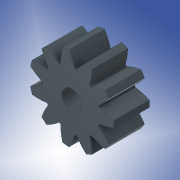
# Autodesk Inventor part: Motor Gear
Saved by Autodesk Inventor 2017 (Build 210142000, 142)
## iProperties
Created: 2017-07-05
Part Number: Motor Gear
Material: ABS Plastic
Document SubType Name: Modeling
Designer: zallen
Density: 1.06 g/cm^3
Appearance: CR Dark Blue
Author: zallen
Autodesk Inventor part; units mm, degrees
ref_plane "YZ Plane" through (0, 0, 0) normal (1, 0, 0) x (0, 1, 0)
ref_plane "XZ Plane" through (0, 0, 0) normal (0, 1, 0) x (-1, 0, 0)
ref_plane "XY Plane" through (0, 0, 0) normal (0, 0, 1) x (1, 0, 0)
sketch "Sketch1" plane through (0, 0, 0) normal (0, 0, 1) x (1, 0, 0)
  circle A0 centre (0, 0) radius 8
  line L0 (0, 0) -> (16, 0) construction
  arc A1 (11.746, 0.9) -> (7.746, 2) centre (5.8068, -12.8741) ccw
  arc A2 (7.746, -2) -> (11.746, -0.9) centre (5.8068, 12.8741) ccw
  arc A3 (7.746, -2) -> (7.746, 2) centre (0, 0) ccw
  arc A4 (11.746, -0.9) -> (11.746, 0.9) centre (-8.2338, 0) ccw
  arc A5 (9.3948, 7.1075) -> (5.435, 5.8703) centre (11.8453, -7.691) ccw
  arc A6 (10.3679, 5.5932) -> (9.3948, 7.1075) centre (-6.9267, -4.4515) ccw
  arc A7 (7.5976, 2.5053) -> (10.3679, 5.5932) centre (-2.0753, 13.9698) ccw
  arc A8 (7.5976, 2.5053) -> (5.435, 5.8703) centre (0, 0) ccw
  arc A9 (4.0608, 11.0584) -> (1.3985, 7.8768) centre (14.123, -0.066) ccw
  arc A10 (5.6981, 10.3106) -> (4.0608, 11.0584) centre (-3.4204, -7.4897) ccw
  arc A11 (5.0371, 6.2151) -> (5.6981, 10.3106) centre (-9.2985, 10.6302) ccw
  arc A12 (5.0371, 6.2151) -> (1.3985, 7.8768) centre (0, 0) ccw
  arc A13 (-2.5625, 11.4983) -> (-3.082, 7.3825) centre (11.9167, 7.5799) ccw
  arc A14 (-0.7808, 11.7545) -> (-2.5625, 11.4983) centre (1.1718, -8.15) ccw
  arc A15 (0.8773, 7.9518) -> (-0.7808, 11.7545) centre (-13.5695, 3.9155) ccw
  arc A16 (0.8773, 7.9518) -> (-3.082, 7.3825) centre (0, 0) ccw
  arc A17 (-8.3721, 8.2876) -> (-6.584, 4.5443) centre (5.927, 12.8193) ccw
  arc A18 (-7.0118, 9.4664) -> (-8.3721, 8.2876) centre (5.392, -6.2227) ccw
  arc A19 (-3.561, 7.1637) -> (-7.0118, 9.4664) centre (-13.5323, -4.0423) ccw
  arc A20 (-3.561, 7.1637) -> (-6.584, 4.5443) centre (0, 0) ccw
  arc A21 (-11.5237, 2.4457) -> (-7.9957, 0.2633) centre (-1.9446, 13.9886) ccw
  arc A22 (-11.0166, 4.1728) -> (-11.5237, 2.4457) centre (7.9002, -2.3197) ccw
  arc A23 (-6.8687, 4.1013) -> (-11.0166, 4.1728) centre (-9.1987, -10.7167) ccw
  arc A24 (-6.8687, 4.1013) -> (-7.9957, 0.2633) centre (0, 0) ccw
  arc A25 (-11.0166, -4.1728) -> (-6.8687, -4.1013) centre (-9.1987, 10.7167) ccw
  arc A26 (-11.5237, -2.4457) -> (-11.0166, -4.1728) centre (7.9002, 2.3197) ccw
  arc A27 (-7.9957, -0.2633) -> (-11.5237, -2.4457) centre (-1.9446, -13.9886) ccw
  arc A28 (-7.9957, -0.2633) -> (-6.8687, -4.1013) centre (0, 0) ccw
  arc A29 (-7.0118, -9.4664) -> (-3.561, -7.1637) centre (-13.5323, 4.0423) ccw
  arc A30 (-8.3721, -8.2876) -> (-7.0118, -9.4664) centre (5.392, 6.2227) ccw
  arc A31 (-6.584, -4.5443) -> (-8.3721, -8.2876) centre (5.927, -12.8193) ccw
  arc A32 (-6.584, -4.5443) -> (-3.561, -7.1637) centre (0, 0) ccw
  arc A33 (-0.7808, -11.7545) -> (0.8773, -7.9518) centre (-13.5695, -3.9155) ccw
  arc A34 (-2.5625, -11.4983) -> (-0.7808, -11.7545) centre (1.1718, 8.15) ccw
  arc A35 (-3.082, -7.3825) -> (-2.5625, -11.4983) centre (11.9167, -7.5799) ccw
  arc A36 (-3.082, -7.3825) -> (0.8773, -7.9518) centre (0, 0) ccw
  arc A37 (5.6981, -10.3106) -> (5.0371, -6.2151) centre (-9.2985, -10.6302) ccw
  arc A38 (4.0608, -11.0584) -> (5.6981, -10.3106) centre (-3.4204, 7.4897) ccw
  arc A39 (1.3985, -7.8768) -> (4.0608, -11.0584) centre (14.123, 0.066) ccw
  arc A40 (1.3985, -7.8768) -> (5.0371, -6.2151) centre (0, 0) ccw
  arc A41 (10.3679, -5.5932) -> (7.5976, -2.5053) centre (-2.0753, -13.9698) ccw
  arc A42 (9.3948, -7.1075) -> (10.3679, -5.5932) centre (-6.9267, 4.4515) ccw
  arc A43 (5.435, -5.8703) -> (9.3948, -7.1075) centre (11.8453, 7.691) ccw
  arc A44 (5.435, -5.8703) -> (7.5976, -2.5053) centre (0, 0) ccw
  point P0 (11.7662, 0)
  point P1 (9.8984, 6.3613)
  point P2 (4.8879, 10.7029)
  point P3 (-1.6745, 11.6465)
  point P4 (-7.7052, 8.8923)
  point P5 (-11.2896, 3.3149)
  point P6 (-11.2896, -3.3149)
  point P7 (-7.7052, -8.8923)
  point P8 (-1.6745, -11.6465)
  point P9 (4.8879, -10.7029)
  point P10 (9.8984, -6.3613)
  dimension "d0" = 16
  dimension "d1" = 16
  dimension "d2" = 15
  dimension "d3" = 4
  dimension "d4" = 2
  dimension "d6" = 1.8
  dimension "d15" = 20
  dimension "d18" = 360
  constraints: 89 point on circle, 44 centre point, 3 symmetric about line, 2 end point, 1 coincident, 1 horizontal, 1 point on line, 150 other
  measures "d1" distance of L0.start L0.end
  measures "d2" radius of A1
  measures "d3" horizontal distance of A1.start A1.end
  measures "d4" distance from line of L0 A1.end
  measures "d6" distance of A2.end A1.start
  measures "d15" radius of A4
extrude "Extrusion1" add sketch "Sketch1" along normal blind 10
sketch "Sketch5" plane through (0, 0, 10) normal (0, 0, 1) x (1, 0, 0)
  circle A0 centre (0, 0) radius 2.75
  dimension "d32" = 5.5
  constraints: 1 centre point, 1 coincident
  measures "d32" diameter of A0
extrude "Extrusion5" cut sketch "Sketch5" against normal through all
body "Solid1"
